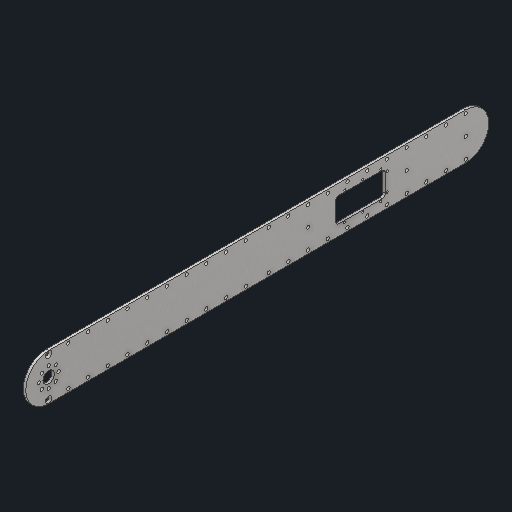
# Autodesk Inventor part: SecondStageArmBar1
Saved by Autodesk Inventor 2025 (Build 290162000, 162)
## iProperties
Created: 2024-01-27
Part Number: SecondStageArmBar1
Material: Aluminum 6061
Document SubType Name: Modeling
Designer: avsar
Density: 2.7 g/cm^3
Appearance: Satin Brushed
Author: avsar
Autodesk Inventor part; units mm, degrees
ref_plane "YZ Plane" through (0, 0, 0) normal (1, 0, 0) x (0, 1, 0)
ref_plane "XZ Plane" through (0, 0, 0) normal (0, 1, 0) x (-1, 0, 0)
ref_plane "XY Plane" through (0, 0, 0) normal (0, 0, 1) x (1, 0, 0)
sketch "Sketch1" plane through (0, 0, 0) normal (1, 0, 0) x (0, 1, 0)
  line L0 (-28, 254) -> (28, 254) construction
  line L1 (28, 254) -> (28, -254)
  line L2 (28, -254) -> (-28, -254) construction
  line L3 (-28, -254) -> (-28, 254)
  line L4 (-28, 254) -> (28, -254) construction
  line L5 (28, 254) -> (-28, -254) construction
  arc A0 (28, 254) -> (-28, 254) centre (0, 254) ccw
  arc A1 (-28, -254) -> (28, -254) centre (0, -254) ccw
  circle A2 centre (0, 254) radius 7
  circle A3 centre (8.4853, 262.4853) radius 2.06
  circle A4 centre (0, 266) radius 2.06
  circle A5 centre (-8.4853, 262.4853) radius 2.06
  circle A6 centre (-12, 254) radius 2.06
  circle A7 centre (0, -254) radius 2.06
  line L6 (8.4853, 262.4853) -> (0, 254) construction
  line L7 (0, 254) -> (0, 261) construction
  circle A8 centre (-8.4853, 245.5147) radius 2.06
  circle A9 centre (0, 242) radius 2.06
  circle A10 centre (8.4853, 245.5147) radius 2.06
  circle A11 centre (12, 254) radius 2.06
  point P0 (0, 0)
  dimension "d2" = 14
  dimension "d0" = 56
  dimension "d1" = 508
  dimension "d3" = 4.12
  dimension "d8" = 360
  dimension "d10" = 4.12
  dimension "d31" = 45
  dimension "d32" = 12
  constraints: 16 end point, 11 centre point, 4 midpoint, 4 point on circle, 4 tangent, 2 coincident, 2 parallel, 1 horizontal, 1 perpendicular, 1 vertical, 1 vertical alignment, 19 other
  measures "d0" distance of L1.end L2.end
  measures "d1" distance of L0.end L1.end
  measures "d3" diameter of A3
  measures "d10" diameter of A7
  measures "d31" angle of L7 L6
  measures "d32" distance of L6.start L6.end
extrude "Extrusion1" add sketch "Sketch1" along normal blind 3
sketch "Sketch2" plane through (3, 0, 0) normal (1, 0, 0) x (0, 0, -1)
  circle A0 centre (-254, 24) radius 2.06
  circle A1 centre (-254, 0) radius 7 construction
  line L0 (254, 28) -> (-254, 28) construction
  circle A2 centre (-230, 24) radius 2.06
  circle A3 centre (-206, 24) radius 2.06
  circle A4 centre (-182, 24) radius 2.06
  circle A5 centre (-158, 24) radius 2.06
  circle A6 centre (-134, 24) radius 2.06
  circle A7 centre (-110, 24) radius 2.06
  circle A8 centre (-86, 24) radius 2.06
  circle A9 centre (-62, 24) radius 2.06
  circle A10 centre (-38, 24) radius 2.06
  circle A11 centre (-14, 24) radius 2.06
  line L1 (0, 28) -> (0, -28) construction
  line L2 (-254, -28) -> (254, -28) construction
  arc A12 (-254, 28) -> (-254, -28) centre (-254, 0) ccw construction
  circle A13 centre (254, 0) radius 2.06 construction
  line L3 (-254, 0) -> (254, 0) construction
  circle A14 centre (254, 24) radius 2.06
  circle A15 centre (230, 24) radius 2.06
  circle A16 centre (206, 24) radius 2.06
  circle A17 centre (182, 24) radius 2.06
  circle A18 centre (158, 24) radius 2.06
  circle A19 centre (134, 24) radius 2.06
  circle A20 centre (110, 24) radius 2.06
  circle A21 centre (86, 24) radius 2.06
  circle A22 centre (62, 24) radius 2.06
  circle A23 centre (38, 24) radius 2.06
  circle A24 centre (14, 24) radius 2.06
  circle A25 centre (-254, -24) radius 2.06
  circle A26 centre (-230, -24) radius 2.06
  circle A27 centre (-206, -24) radius 2.06
  circle A28 centre (-182, -24) radius 2.06
  circle A29 centre (-158, -24) radius 2.06
  circle A30 centre (-134, -24) radius 2.06
  circle A31 centre (-110, -24) radius 2.06
  circle A32 centre (-86, -24) radius 2.06
  circle A33 centre (-62, -24) radius 2.06
  circle A34 centre (-38, -24) radius 2.06
  circle A35 centre (-14, -24) radius 2.06
  circle A36 centre (254, -24) radius 2.06
  circle A37 centre (230, -24) radius 2.06
  circle A38 centre (206, -24) radius 2.06
  circle A39 centre (182, -24) radius 2.06
  circle A40 centre (158, -24) radius 2.06
  circle A41 centre (134, -24) radius 2.06
  circle A42 centre (86, -24) radius 2.06
  circle A43 centre (62, -24) radius 2.06
  circle A44 centre (38, -24) radius 2.06
  circle A45 centre (14, -24) radius 2.06
  circle A46 centre (110, -24) radius 2.06
  point P0 (0, 0)
  dimension "d20" = 4.12
  dimension "d21" = 4
  dimension "d24" = 24
  constraints: 44 centre point, 33 symmetric about line, 4 end point, 2 horizontal, 2 midpoint, 1 vertical alignment, 53 other
  measures "d20" diameter of A0
  measures "d21" distance from line of L0 A0.centre
  measures "d24" distance of A0.centre A2.centre
extrude "Extrusion2" cut sketch "Sketch2" against normal through all
sketch "Sketch5" plane through (3, 0, 0) normal (1, 0, 0) x (0, 0, -1)
  circle A0 centre (254, 0) radius 2.06 construction
  line L0 (254, 0) -> (110.517, 0) construction
  line L1 (110.517, 0) -> (106.517, 0) construction
  line L2 (106.517, 0) -> (106.517, -17) construction
  circle A1 centre (106.517, -17) radius 1.3
  circle A2 centre (128.517, -17) radius 1.3
  circle A3 centre (150.517, -17) radius 1.3
  circle A4 centre (106.517, 17) radius 1.3
  circle A5 centre (128.517, 17) radius 1.3
  circle A6 centre (150.517, 17) radius 1.3
  circle A7 centre (158.317, -11) radius 1.3
  circle A8 centre (158.317, 11) radius 1.3
  line L3 (152.017, -14.5) -> (99.517, -14.5) construction
  line L4 (96.017, -11) -> (96.017, 11) construction
  line L5 (99.517, 14.5) -> (152.017, 14.5) construction
  line L6 (155.517, 11) -> (155.517, -11) construction
  arc A9 (99.517, 14.5) -> (96.017, 11) centre (99.517, 11) ccw construction
  arc A10 (96.017, -11) -> (99.517, -14.5) centre (99.517, -11) ccw construction
  arc A11 (152.017, -14.5) -> (155.517, -11) centre (152.017, -11) ccw construction
  arc A12 (155.517, 11) -> (152.017, 14.5) centre (152.017, 11) ccw construction
  line L7 (95.517, 11) -> (95.517, -11)
  arc A13 (95.517, -11) -> (99.517, -15) centre (99.517, -11) ccw
  line L8 (99.517, -15) -> (152.017, -15)
  arc A14 (152.017, -15) -> (156.017, -11) centre (152.017, -11) ccw
  line L9 (156.017, -11) -> (156.017, 11)
  arc A15 (156.017, 11) -> (152.017, 15) centre (152.017, 11) ccw
  line L10 (152.017, 15) -> (99.517, 15)
  arc A16 (99.517, 15) -> (95.517, 11) centre (99.517, 11) ccw
  point P0 (0, 0)
  point P1 (155.517, -14.5)
  point P2 (96.017, 14.5)
  point P3 (155.517, 14.5)
  dimension "d37" = 143.483
  dimension "d38" = 4
  dimension "d39" = 17
  dimension "d40" = 2.6
  dimension "d41" = 2.6
  dimension "d42" = 22
  dimension "d43" = 2.6
  dimension "d44" = 22
  dimension "d45" = 2.6
  dimension "d47" = 7.8
  dimension "d48" = 11
  dimension "d49" = 14.5
  dimension "d50" = 5
  dimension "d51" = 29
  dimension "d52" = 59.5
  dimension "d53" = 3.5
  dimension "d54" = 3.5
  dimension "d55" = 0.5
  constraints: 22 end point, 16 centre point, 16 point on circle, 8 tangent, 6 point on line, 5 symmetric about line, 4 parallel, 3 horizontal, 3 perpendicular, 2 coincident, 2 equal radius, 2 horizontal alignment, 11 other
  measures "d37" distance of L0.start L0.end
  measures "d38" distance of L0.end L1.end
  measures "d39" distance of L1.end L2.end
  measures "d40" diameter of A1
  measures "d41" diameter of A2
  measures "d42" distance of L2.end A2.centre
  measures "d43" diameter of A3
  measures "d44" distance of A2.centre A3.centre
  measures "d45" diameter of A7
  measures "d47" horizontal distance of A7.centre A3.centre
  measures "d48" distance from line of L0 A7.centre
  measures "d49" distance from line of L0 point (155.517, -14.5)
  measures "d50" horizontal distance of A3.centre point (155.517, -14.5)
  measures "d51" distance of point (155.517, 14.5) point (155.517, -14.5)
  measures "d52" distance of point (96.017, 14.5) point (155.517, 14.5)
  measures "d53" radius of A9
  measures "d54" radius of A10
  measures "d55" radial gap between concentric circles of A9 A16
extrude "Extrusion4" cut sketch "Sketch5" against normal through all
sketch "Sketch6" plane through (3, 0, 0) normal (1, 0, 0) x (0, 0, -1)
  circle A0 centre (182, 0) radius 2.06
  circle A1 centre (254, 0) radius 2.06 construction
  circle A2 centre (62, 0) radius 2.06
  point P0 (0, 0)
  dimension "d58" = 4.12
  dimension "d59" = 72
  dimension "d60" = 4.12
  dimension "d61" = 120
  constraints: 2 centre point, 2 horizontal alignment
  measures "d58" diameter of A0
  measures "d59" distance of A1.centre A0.centre
  measures "d60" diameter of A2
  measures "d61" distance of A2.centre A0.centre
extrude "Extrusion5" cut sketch "Sketch6" against normal through all
hole "Hole1" at (3, 24, 254) at (3, -24, 254) direction (-1, 0, 0) diameter 4.12 end through all countersink diameter 8 countersink angle 90
equation "\"d41\" = d40"
equation "\"d43\" = d40"
body "Solid1"
